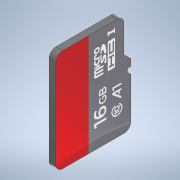
# Autodesk Inventor part: microsd
Saved by Autodesk Inventor 2021.2 (Build 252289000, 289)
## iProperties
Created: 2022-12-19
Part Number: microsd
Material: 일반
Document SubType Name: Modeling
Designer: dbstj
Density: 1 g/cm^3
Appearance: 기본값
Author: dbstj
Autodesk Inventor part; units mm, degrees
ref_plane "YZ Plane" through (0, 0, 0) normal (1, 0, 0) x (0, 1, 0)
ref_plane "XZ Plane" through (0, 0, 0) normal (0, 1, 0) x (-1, 0, 0)
ref_plane "XY Plane" through (0, 0, 0) normal (0, 0, 1) x (1, 0, 0)
sketch "스케치1" plane through (0, 0, 0) normal (1, 0, 0) x (0, 1, 0)
  line L0 (0, 0) -> (15, 0)
  line L1 (15, 0) -> (15, -11)
  line L2 (15, -11) -> (0, -11)
  line L3 (0, -11) -> (0, 0)
  line L4 (15, -11) -> (8.9773, -11)
  line L5 (10, -9.9773) -> (15, -9.9773)
  line L6 (15, -9.9773) -> (15, -11)
  line L7 (0, -11) -> (5, -11)
  line L8 (0, -10) -> (0, -11)
  line L9 (5, -11) -> (7, -11)
  line L10 (7, -11) -> (8, -11)
  line L11 (8, -11) -> (8, -10.5)
  line L12 (8.9773, -11) -> (10, -9.9773)
  line L13 (8.9773, -11) -> (10.4236, -11) construction
  line L14 (7, -11) -> (7.5, -10.5)
  line L15 (8, -10.5) -> (7.5, -10.5)
  dimension "d0" = 15
  dimension "d1" = 11
  dimension "d8" = 45
  dimension "d9" = 5
  constraints: 32 end point, 7 horizontal, 3 parallel, 3 perpendicular, 1 equal length
  measures "d0" distance of L1.end L2.end
  measures "d1" distance of L0.end L1.end
  measures "d8" angle of L13 L12
  measures "d9" distance of L5.start L5.end
extrude "돌출1" add sketch "스케치1" along normal blind 1 contours L0 L1 L5 L12 L2 L11 L15 L14 L3
fillet "모깎기1" radius 1 4 edges at (0.5, 15, -9.9773) (0.5, 15, 0) (0.5, 0, -11) (0.5, 0, 0)
sketch "스케치2" plane through (1, 0, 0) normal (1, 0, 0) x (0, 0, -1)
  arc A0 (0, 1) -> (1, 0) centre (1, 1) ccw projected
  line L0 (1, 0) -> (10, 0) projected
  arc A1 (10, 0) -> (11, 1) centre (10, 1) ccw projected
  line L1 (11, 1) -> (11, 7) projected
  line L2 (11, 7) -> (10.5, 7.5) projected
  line L3 (10.5, 7.5) -> (10.5, 8) projected
  line L4 (10.5, 8) -> (11, 8) projected
  line L5 (11, 8) -> (11, 8.9773) projected
  line L6 (11, 8.9773) -> (9.9773, 10) projected
  line L7 (9.9773, 10) -> (9.9773, 14) projected
  arc A2 (9.9773, 14) -> (8.9773, 15) centre (8.9773, 14) ccw projected
  line L8 (8.9773, 15) -> (1, 15) projected
  arc A3 (1, 15) -> (0, 14) centre (1, 14) ccw projected
  line L9 (0, 14) -> (0, 1) projected
  line L10 (-0.1139, -0.2414) -> (-0.1139, 15.1589) construction
  line L11 (-0.1139, 15.1589) -> (11.0874, 15.1589) construction
  line L12 (11.0874, 15.1589) -> (11.0874, -0.2414) construction
  line L13 (11.0874, -0.2414) -> (-0.1139, -0.2414) construction
  point P0 (0, 0)
  constraints: 2 other
decal "전사1"
